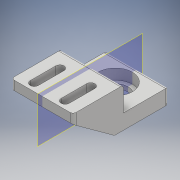
# Autodesk Inventor part: Estrutura - Rolamento Esquerdo
Saved by Autodesk Inventor 2017 (Build 210142000, 142)
## iProperties
Created: 2020-08-07
Part Number: Estrutura - Rolamento Esquerdo
Material: Generic
Document SubType Name: Modeling
Designer: ale
Density: 1 g/cm^3
Appearance: Default
Author: ale
Autodesk Inventor part; units mm, degrees
ref_plane "YZ Plane" through (0, 0, 0) normal (1, 0, 0) x (0, 1, 0)
ref_plane "XZ Plane" through (0, 0, 0) normal (0, 1, 0) x (-1, 0, 0)
ref_plane "XY Plane" through (0, 0, 0) normal (0, 0, 1) x (1, 0, 0)
sketch "Sketch1" plane through (0, 0, 0) normal (0, 0, 1) x (1, 0, 0)
  line L0 (-20.5, 15) -> (20.5, 15)
  line L1 (20.5, 15) -> (20.5, -15)
  line L2 (20.5, -15) -> (-20.5, -15)
  line L3 (-20.5, -15) -> (-20.5, 15)
  line L4 (-20.5, 15) -> (20.5, -15) construction
  line L5 (20.5, 15) -> (-20.5, -15) construction
  circle A0 centre (0, 0) radius 11.35
  line L6 (16.5, 15) -> (16.5, -15)
  dimension "d0" = 41
  dimension "d1" = 30
  dimension "d2" = 22.7
  dimension "d4" = 4
  constraints: 14 end point, 3 parallel, 2 midpoint, 1 centre point, 1 coincident, 1 horizontal, 1 perpendicular
  measures "d0" distance of L1.end L2.end
  measures "d1" distance of L0.end L1.end
  measures "d2" diameter of A0
  measures "d4" distance between parallel lines of L1 L6
extrude "Extrusion3" add sketch "Sketch1" along normal blind 10
sketch "Sketch3" plane through (0, 0, 0) normal (0, 0, -1) x (-1, 0, 0)
  circle A0 centre (0, 0) radius 11.35
  circle A1 centre (0, 0) radius 11.35 projected
  circle A2 centre (0, 0) radius 8.5
  dimension "d18" = 17
  constraints: 2 centre point, 2 coincident
  measures "d18" diameter of A2
extrude "Extrusion4" add sketch "Sketch3" against normal blind 3
sketch "Sketch4" plane through (-20.5, -15, 0) normal (0, -1, 0) x (1, 0, 0)
  line L0 (0, 0) -> (0, 10) projected
  line L1 (0, 0) -> (41, 0)
  line L2 (41, 0) -> (41, 20)
  line L3 (41, 20) -> (0, 20)
  line L4 (0, 20) -> (0, 0)
  point P0 (20.5, 0)
  dimension "d21" = 20
  dimension "d22" = 41
  constraints: 8 end point, 2 parallel, 1 horizontal, 1 perpendicular
  measures "d21" distance between parallel lines of L1 L3
  measures "d22" distance between parallel lines of L2 L4
extrude "Extrusion5" add sketch "Sketch4" along normal blind 6
sketch "Sketch5" plane through (-20.5, -15, 20) normal (0, 0, 1) x (1, 0, 0)
  line L0 (0, 30) -> (0, 0) projected
  line L1 (0, 0) -> (41, 0)
  line L2 (41, 0) -> (41, -33.5)
  line L3 (41, -33.5) -> (0, -33.5)
  line L4 (0, -33.5) -> (0, 0)
  point P0 (20.5, 15)
  dimension "d25" = 33.5
  dimension "d69" = 41
  constraints: 8 end point, 2 parallel, 1 horizontal, 1 perpendicular
  measures "d25" distance of L1.end L2.end
  measures "d69" distance between parallel lines of L2 L4
extrude "Extrusion6" add sketch "Sketch5" along normal blind 6
sketch "Sketch13" plane through (20.5, 15, 10) normal (1, 0, 0) x (0, 0, -1)
  line L0 (-10, -63.5) -> (-16, -63.5) projected
  line L1 (-10, -63.5) -> (-10, -36) projected
  line L2 (-16, -63.5) -> (-10, -63.5)
  line L3 (-10, -63.5) -> (10, -36)
  line L4 (10, -36) -> (10, -30)
  line L5 (0, 0) -> (0, -30) projected
  line L6 (10, -30) -> (-16, -30)
  line L7 (-16, -30) -> (-16, -63.5) projected
  line L8 (-16, -30) -> (-16, -63.5)
  point P0 (10, -15)
  point P1 (-16, -56.5)
  constraints: 10 end point, 2 perpendicular, 1 collinear, 1 parallel
extrude "Extrusion10" add sketch "Sketch13" against normal blind 2
ref_plane "Work Plane1" through (0, 15, 0) normal (-1, 0, 0) x (0, 0, 1)
mirror "Mirror1" about plane through (0, 15, 0) normal (-1, 0, 0) of "Extrusion10"
fillet "Fillet2" radius 2 4 edges at (20.5, 15, 5) (-20.5, 15, 5) (0, 15, 10) (0, 15, 0)
sketch "Sketch15" plane through (-20.5, -15, 26) normal (0, 0, 1) x (1, 0, 0)
  arc A0 (13, -11.5) -> (7.5, -11.5) centre (10.25, -11.5) ccw
  line L0 (2, -33.5) -> (39, -33.5) projected
  line L1 (0, -2) -> (0, -31.5) projected
  arc A1 (7.5, -28.5) -> (13, -28.5) centre (10.25, -28.5) ccw
  line L2 (7.5, -11.5) -> (7.5, -28.5)
  line L3 (13, -11.5) -> (13, -28.5)
  line L4 (20.5, -33.5) -> (20.5, -2)
  arc A2 (33.5, -11.5) -> (28, -11.5) centre (30.75, -11.5) ccw
  arc A3 (28, -28.5) -> (33.5, -28.5) centre (30.75, -28.5) ccw
  line L5 (33.5, -11.5) -> (33.5, -28.5)
  line L6 (28, -11.5) -> (28, -28.5)
  point P0 (20.5, 15)
  dimension "d74" = 5.5
  dimension "d75" = 22
  dimension "d76" = 10.25
  dimension "d77" = 5.5
  dimension "d78" = 5
  dimension "d79" = 10.25
  constraints: 10 end point, 8 point on circle, 6 symmetric about line, 4 centre point, 2 tangent, 2 vertical, 1 midpoint, 1 parallel, 2 other
  measures "d74" diameter of A0
  measures "d75" distance from line of L0 A0.centre
  measures "d76" distance from line of L1 A0.centre
  measures "d77" diameter of A1
  measures "d78" distance from line of L0 A1.centre
  measures "d79" distance from line of L1 A1.centre
extrude "Extrusion11" cut sketch "Sketch15" against normal through all
body "Solid2"
